Autodesk Inventor part; units mm, degrees
(part 2 of 3)
  line L262 (-273.1274, 163.0972) -> (-274.8776, 163.4871)
  line L263 (-274.8776, 163.4871) -> (-276.0608, 161.4819)
  line L264 (-276.0608, 161.4819) -> (-274.8734, 160.1383)
  line L265 (-274.8734, 160.1383) -> (-275.2904, 159.4316)
  line L266 (-275.5866, 163.6472) -> (-278.54, 164.2936)
  line L267 (-278.54, 164.2936) -> (-276.5438, 162.0252)
  line L268 (-276.5438, 162.0252) -> (-275.5866, 163.6472)
  line L269 (-271.6069, 165.6091) -> (-276.1953, 168.4149)
  line L270 (-276.1953, 168.4149) -> (-277.263, 166.669)
  line L271 (-277.263, 166.669) -> (-277.8787, 167.0455)
  line L272 (-277.8787, 167.0455) -> (-275.3204, 171.229)
  line L273 (-275.3204, 171.229) -> (-274.7047, 170.8525)
  line L274 (-274.7047, 170.8525) -> (-275.7724, 169.1065)
  line L275 (-275.7724, 169.1065) -> (-271.184, 166.3007)
  line L276 (-271.184, 166.3007) -> (-271.6069, 165.6091)
  spline S181 degree 2 poles (-268.782, 169.9517) (-269.136, 169.3919) (-269.8667, 168.7544) (-270.2531, 168.5133) knots 0 0 0 1 2 2 2
  line L277 (-270.2531, 168.5133) -> (-271.1138, 169.0576)
  line L278 (-271.1138, 169.0576) -> (-271.0821, 169.1077)
  spline S182 degree 2 poles (-271.0821, 169.1077) (-270.5505, 169.2453) (-269.6579, 169.8799) (-269.407, 170.2768) knots 0 0 0 1 2 2 2
  spline S183 degree 2 poles (-269.407, 170.2768) (-269.0476, 170.845) (-269.1525, 171.7243) (-269.541, 171.97) knots 0 0 0 1 2 2 2
  spline S184 degree 2 poles (-269.541, 171.97) (-269.8502, 172.1655) (-270.4275, 172.1036) (-270.7323, 171.8343) knots 0 0 0 1 2 2 2
  spline S185 degree 2 poles (-270.7323, 171.8343) (-270.9497, 171.6384) (-271.2926, 171.2996) (-271.5554, 171.0506) knots 0 0 0 1 2 2 2
  spline S186 degree 2 poles (-271.5554, 171.0506) (-271.7955, 170.8281) (-272.2755, 170.5408) (-272.5498, 170.4862) knots 0 0 0 1 2 2 2
  spline S187 degree 2 poles (-272.5498, 170.4862) (-272.8215, 170.4358) (-273.392, 170.5509) (-273.6929, 170.7412) knots 0 0 0 1 2 2 2
  spline S188 degree 2 poles (-273.6929, 170.7412) (-274.3196, 171.1375) (-274.5494, 172.6515) (-274.0712, 173.4077) knots 0 0 0 1 2 2 2
  spline S189 degree 2 poles (-274.0712, 173.4077) (-273.7964, 173.8422) (-273.139, 174.5026) (-272.7673, 174.7296) knots 0 0 0 1 2 2 2
  line L279 (-272.7673, 174.7296) -> (-271.9485, 174.2118)
  line L280 (-271.9485, 174.2118) -> (-271.9802, 174.1617)
  spline S190 degree 2 poles (-271.9802, 174.1617) (-272.3617, 174.0578) (-273.182, 173.5004) (-273.4489, 173.0785) knots 0 0 0 1 2 2 2
  spline S191 degree 2 poles (-273.4489, 173.0785) (-273.7501, 172.6022) (-273.6756, 171.7304) (-273.3121, 171.5005) knots 0 0 0 1 2 2 2
  spline S192 degree 2 poles (-273.3121, 171.5005) (-272.9862, 171.2944) (-272.3784, 171.3955) (-272.0845, 171.6659) knots 0 0 0 1 2 2 2
  spline S193 degree 2 poles (-272.0845, 171.6659) (-271.8887, 171.8462) (-271.3393, 172.3819) (-271.1445, 172.5512) knots 0 0 0 1 2 2 2
  spline S194 degree 2 poles (-271.1445, 172.5512) (-270.6461, 172.9788) (-269.6783, 173.057) (-269.1979, 172.7531) knots 0 0 0 1 2 2 2
  spline S195 degree 2 poles (-269.1979, 172.7531) (-268.8929, 172.5602) (-268.4639, 171.9439) (-268.3992, 171.593) knots 0 0 0 1 2 2 2
  spline S196 degree 2 poles (-268.3992, 171.593) (-268.3294, 171.2038) (-268.4834, 170.4239) (-268.782, 169.9517) knots 0 0 0 1 2 2 2
  line L281 (-267.6393, 171.9664) -> (-271.6185, 177.0265)
  line L282 (-271.6185, 177.0265) -> (-271.0719, 177.8622)
  line L283 (-271.0719, 177.8622) -> (-264.8413, 176.2439)
  line L284 (-264.8413, 176.2439) -> (-265.3095, 175.5282)
  line L285 (-265.3095, 175.5282) -> (-267.0398, 175.9985)
  line L286 (-267.0398, 175.9985) -> (-268.3143, 174.05)
  line L287 (-268.3143, 174.05) -> (-267.1901, 172.6531)
  line L288 (-267.1901, 172.6531) -> (-267.6393, 171.9664)
  line L289 (-267.7407, 176.1912) -> (-270.6611, 176.9732)
  line L290 (-270.6611, 176.9732) -> (-268.7717, 174.615)
  line L291 (-268.7717, 174.615) -> (-267.7407, 176.1912)
  spline S197 degree 2 poles (-266.5204, 183.3958) (-265.9906, 183.4543) (-264.7926, 183.1067) (-264.1628, 182.6789) knots 0 0 0 1 2 2 2
  spline S198 degree 2 poles (-264.1628, 182.6789) (-263.5494, 182.2623) (-262.7668, 181.2766) (-262.6315, 180.7545) knots 0 0 0 1 2 2 2
  spline S199 degree 2 poles (-262.6315, 180.7545) (-262.4909, 180.2048) (-262.7138, 179.1551) (-263.0499, 178.6603) knots 0 0 0 1 2 2 2
  spline S200 degree 2 poles (-263.0499, 178.6603) (-263.3971, 178.1492) (-264.3002, 177.5674) (-264.8423, 177.4994) knots 0 0 0 1 2 2 2
  spline S201 degree 2 poles (-264.8423, 177.4994) (-265.3748, 177.4368) (-266.5714, 177.7954) (-267.193, 178.2176) knots 0 0 0 1 2 2 2
  spline S202 degree 2 poles (-267.193, 178.2176) (-267.8268, 178.6481) (-268.578, 179.6184) (-268.7284, 180.1448) knots 0 0 0 1 2 2 2
  spline S203 degree 2 poles (-268.7284, 180.1448) (-268.8638, 180.667) (-268.6531, 181.725) (-268.3087, 182.2321) knots 0 0 0 1 2 2 2
  spline S204 degree 2 poles (-268.3087, 182.2321) (-267.9587, 182.7473) (-267.0378, 183.3289) (-266.5204, 183.3958) knots 0 0 0 1 2 2 2
  spline S205 degree 2 poles (-264.6378, 181.9797) (-265.1367, 182.3185) (-266.0567, 182.6267) (-266.4436, 182.6026) knots 0 0 0 1 2 2 2
  spline S206 degree 2 poles (-266.4436, 182.6026) (-266.8414, 182.58) (-267.4864, 182.1935) (-267.7252, 181.8418) knots 0 0 0 1 2 2 2
  spline S207 degree 2 poles (-267.7252, 181.8418) (-267.9724, 181.4778) (-268.0911, 180.7577) (-267.9628, 180.3658) knots 0 0 0 1 2 2 2
  spline S208 degree 2 poles (-267.9628, 180.3658) (-267.8413, 179.9905) (-267.2088, 179.2501) (-266.718, 178.9168) knots 0 0 0 1 2 2 2
  spline S209 degree 2 poles (-266.718, 178.9168) (-265.7244, 178.2419) (-264.1027, 178.3595) (-263.6278, 179.0588) knots 0 0 0 1 2 2 2
  spline S210 degree 2 poles (-263.6278, 179.0588) (-263.1529, 179.7581) (-263.6441, 181.3048) (-264.6378, 181.9797) knots 0 0 0 1 2 2 2
  spline S211 degree 2 poles (-259.7955, 183.3604) (-260.1062, 182.9202) (-260.7982, 182.4284) (-261.1909, 182.3607) knots 0 0 0 1 2 2 2
  spline S212 degree 2 poles (-261.1909, 182.3607) (-261.6346, 182.2806) (-262.5127, 182.5797) (-263.0458, 182.9559) knots 0 0 0 1 2 2 2
  line L292 (-263.0458, 182.9559) -> (-266.1555, 185.1508)
  line L293 (-266.1555, 185.1508) -> (-265.6881, 185.8131)
  line L294 (-265.6881, 185.8131) -> (-262.5783, 183.6183)
  spline S213 degree 2 poles (-262.5783, 183.6183) (-262.231, 183.3731) (-261.6998, 183.1313) (-261.4216, 183.1226) knots 0 0 0 1 2 2 2
  spline S214 degree 2 poles (-261.4216, 183.1226) (-261.1256, 183.1133) (-260.5947, 183.4283) (-260.3609, 183.7595) knots 0 0 0 1 2 2 2
  spline S215 degree 2 poles (-260.3609, 183.7595) (-260.1415, 184.0705) (-260.0054, 184.7005) (-260.1132, 184.9763) knots 0 0 0 1 2 2 2
  spline S216 degree 2 poles (-260.1132, 184.9763) (-260.2147, 185.2355) (-260.6164, 185.6521) (-260.9516, 185.8887) knots 0 0 0 1 2 2 2
  line L295 (-260.9516, 185.8887) -> (-264.0775, 188.095)
  line L296 (-264.0775, 188.095) -> (-263.6101, 188.7573)
  line L297 (-263.6101, 188.7573) -> (-260.5003, 186.5625)
  spline S217 degree 2 poles (-260.5003, 186.5625) (-259.9793, 186.1947) (-259.3844, 185.4602) (-259.3181, 185.0141) knots 0 0 0 1 2 2 2
  spline S218 degree 2 poles (-259.3181, 185.0141) (-259.2521, 184.6105) (-259.4706, 183.8208) (-259.7955, 183.3604) knots 0 0 0 1 2 2 2
  line L298 (-255.3693, 189.7045) -> (-255.9067, 188.9707)
  line L299 (-255.9067, 188.9707) -> (-261.7448, 189.9005)
  line L300 (-261.7448, 189.9005) -> (-257.5013, 186.7931)
  line L301 (-257.5013, 186.7931) -> (-257.9481, 186.1829)
  line L302 (-257.9481, 186.1829) -> (-262.8697, 189.7868)
  line L303 (-262.8697, 189.7868) -> (-262.1892, 190.7161)
  line L304 (-262.1892, 190.7161) -> (-256.8411, 189.8449)
  line L305 (-256.8411, 189.8449) -> (-260.7377, 192.6983)
  line L306 (-260.7377, 192.6983) -> (-260.2908, 193.3085)
  line L307 (-260.2908, 193.3085) -> (-255.3693, 189.7045)
  line L308 (-253.3463, 192.3891) -> (-254.7684, 190.502)
  line L309 (-254.7684, 190.502) -> (-255.2658, 190.8768)
  line L310 (-255.2658, 190.8768) -> (-254.7987, 191.4967)
  line L311 (-254.7987, 191.4967) -> (-258.6755, 194.4181)
  line L312 (-258.6755, 194.4181) -> (-259.1426, 193.7983)
  line L313 (-259.1426, 193.7983) -> (-259.64, 194.1731)
  line L314 (-259.64, 194.1731) -> (-258.218, 196.0602)
  line L315 (-258.218, 196.0602) -> (-257.7205, 195.6853)
  line L316 (-257.7205, 195.6853) -> (-258.1876, 195.0655)
  line L317 (-258.1876, 195.0655) -> (-254.3108, 192.1441)
  line L318 (-254.3108, 192.1441) -> (-253.8438, 192.7639)
  line L319 (-253.8438, 192.7639) -> (-253.3463, 192.3891)
  spline S219 degree 2 poles (-252.2013, 198.8575) (-251.5411, 198.3456) (-250.8937, 196.9864) (-250.9452, 196.307) knots 0 0 0 1 2 2 2
  spline S220 degree 2 poles (-250.9452, 196.307) (-250.9995, 195.761) (-251.4279, 194.886) (-251.8823, 194.3) knots 0 0 0 1 2 2 2
  line L320 (-251.8823, 194.3) -> (-252.7427, 193.1907)
  line L321 (-252.7427, 193.1907) -> (-257.563, 196.9289)
  line L322 (-257.563, 196.9289) -> (-256.7117, 198.0266)
  spline S221 degree 2 poles (-256.7117, 198.0266) (-256.1846, 198.7063) (-255.3816, 199.3222) (-254.9899, 199.4563) knots 0 0 0 1 2 2 2
  spline S222 degree 2 poles (-254.9899, 199.4563) (-254.3208, 199.6818) (-252.9044, 199.4028) (-252.2013, 198.8575) knots 0 0 0 1 2 2 2
  spline S223 degree 2 poles (-252.7271, 198.1956) (-253.2818, 198.6258) (-254.3517, 198.8675) (-254.8561, 198.6769) knots 0 0 0 1 2 2 2
  spline S224 degree 2 poles (-254.8561, 198.6769) (-255.2084, 198.5373) (-255.7965, 198.0613) (-256.1328, 197.6277) knots 0 0 0 1 2 2 2
  line L323 (-256.1328, 197.6277) -> (-256.5115, 197.1394)
  line L324 (-256.5115, 197.1394) -> (-252.8005, 194.2615)
  line L325 (-252.8005, 194.2615) -> (-252.4219, 194.7497)
  spline S225 degree 2 poles (-252.4219, 194.7497) (-252.0916, 195.1755) (-251.7285, 195.9261) (-251.7091, 196.3302) knots 0 0 0 1 2 2 2
  spline S226 degree 2 poles (-251.7091, 196.3302) (-251.6752, 196.8418) (-252.1646, 197.7594) (-252.7271, 198.1956) knots 0 0 0 1 2 2 2
  line L326 (-247.9163, 199.3374) -> (-249.3901, 197.4905)
  line L327 (-249.3901, 197.4905) -> (-249.877, 197.879)
  line L328 (-249.877, 197.879) -> (-249.3929, 198.4856)
  line L329 (-249.3929, 198.4856) -> (-253.1872, 201.5133)
  line L330 (-253.1872, 201.5133) -> (-253.6713, 200.9067)
  line L331 (-253.6713, 200.9067) -> (-254.1582, 201.2952)
  line L332 (-254.1582, 201.2952) -> (-252.6844, 203.1421)
  line L333 (-252.6844, 203.1421) -> (-252.1975, 202.7537)
  line L334 (-252.1975, 202.7537) -> (-252.6816, 202.147)
  line L335 (-252.6816, 202.147) -> (-248.8873, 199.1193)
  line L336 (-248.8873, 199.1193) -> (-248.4032, 199.7259)
  line L337 (-248.4032, 199.7259) -> (-247.9163, 199.3374)
  spline S227 degree 2 poles (-246.1272, 201.3672) (-246.5467, 200.8545) (-247.3494, 200.3106) (-247.7623, 200.1183) knots 0 0 0 1 2 2 2
  line L338 (-247.7623, 200.1183) -> (-248.5504, 200.7631)
  line L339 (-248.5504, 200.7631) -> (-248.5128, 200.809)
  spline S228 degree 2 poles (-248.5128, 200.809) (-247.9685, 200.881) (-247.0054, 201.4023) (-246.708, 201.7658) knots 0 0 0 1 2 2 2
  spline S229 degree 2 poles (-246.708, 201.7658) (-246.2823, 202.2861) (-246.2795, 203.1716) (-246.6353, 203.4627) knots 0 0 0 1 2 2 2
  spline S230 degree 2 poles (-246.6353, 203.4627) (-246.9184, 203.6944) (-247.4989, 203.7031) (-247.8342, 203.4729) knots 0 0 0 1 2 2 2
  spline S231 degree 2 poles (-247.8342, 203.4729) (-248.0738, 203.3049) (-248.4554, 203.0103) (-248.7465, 202.795) knots 0 0 0 1 2 2 2
  spline S232 degree 2 poles (-248.7465, 202.795) (-249.0119, 202.6034) (-249.5232, 202.3766) (-249.8021, 202.3558) knots 0 0 0 1 2 2 2
  spline S233 degree 2 poles (-249.8021, 202.3558) (-250.0779, 202.3387) (-250.6302, 202.5224) (-250.9057, 202.7478) knots 0 0 0 1 2 2 2
  spline S234 degree 2 poles (-250.9057, 202.7478) (-251.4796, 203.2173) (-251.5237, 204.748) (-250.9571, 205.4405) knots 0 0 0 1 2 2 2
  spline S235 degree 2 poles (-250.9571, 205.4405) (-250.6315, 205.8384) (-249.8987, 206.414) (-249.5022, 206.5941) knots 0 0 0 1 2 2 2
  line L340 (-249.5022, 206.5941) -> (-248.7523, 205.9806)
  line L341 (-248.7523, 205.9806) -> (-248.7899, 205.9347)
  spline S236 degree 2 poles (-248.7899, 205.9347) (-249.1812, 205.878) (-250.0632, 205.4245) (-250.3794, 205.0381) knots 0 0 0 1 2 2 2
  spline S237 degree 2 poles (-250.3794, 205.0381) (-250.7362, 204.6019) (-250.7683, 203.7276) (-250.4354, 203.4552) knots 0 0 0 1 2 2 2
  spline S238 degree 2 poles (-250.4354, 203.4552) (-250.137, 203.211) (-249.5214, 203.2375) (-249.1969, 203.4701) knots 0 0 0 1 2 2 2
  spline S239 degree 2 poles (-249.1969, 203.4701) (-248.9805, 203.6252) (-248.3701, 204.0902) (-248.1562, 204.2346) knots 0 0 0 1 2 2 2
  spline S240 degree 2 poles (-248.1562, 204.2346) (-247.6095, 204.5984) (-246.6394, 204.5583) (-246.1995, 204.1983) knots 0 0 0 1 2 2 2
  spline S241 degree 2 poles (-246.1995, 204.1983) (-245.9202, 203.9698) (-245.5693, 203.3059) (-245.5477, 202.9497) knots 0 0 0 1 2 2 2
  spline S242 degree 2 poles (-245.5477, 202.9497) (-245.5258, 202.5549) (-245.7735, 201.7995) (-246.1272, 201.3672) knots 0 0 0 1 2 2 2
  spline S243 degree 2 poles (-241.7417, 209.8177) (-241.3851, 209.5121) (-240.9834, 208.7578) (-240.9512, 208.3851) knots 0 0 0 1 2 2 2
  spline S244 degree 2 poles (-240.9512, 208.3851) (-240.9142, 207.9953) (-241.1366, 207.2876) (-241.4036, 206.976) knots 0 0 0 1 2 2 2
  spline S245 degree 2 poles (-241.4036, 206.976) (-241.6706, 206.6645) (-242.3215, 206.3304) (-242.6989, 206.3153) knots 0 0 0 1 2 2 2
  spline S246 degree 2 poles (-242.6989, 206.3153) (-243.1563, 206.2906) (-244.2324, 206.7441) (-244.848, 207.2717) knots 0 0 0 1 2 2 2
  spline S247 degree 2 poles (-244.848, 207.2717) (-245.4523, 207.7895) (-246.2122, 208.8704) (-246.3506, 209.4382) knots 0 0 0 1 2 2 2
  spline S248 degree 2 poles (-246.3506, 209.4382) (-246.4879, 209.9921) (-246.2001, 211.1255) (-245.753, 211.6473) knots 0 0 0 1 2 2 2
  spline S249 degree 2 poles (-245.753, 211.6473) (-245.6211, 211.8012) (-245.3594, 212.0457) (-245.2388, 212.1181) knots 0 0 0 1 2 2 2
  line L342 (-245.2388, 212.1181) -> (-244.642, 211.6066)
  line L343 (-244.642, 211.6066) -> (-244.6645, 211.5804)
  spline S250 degree 2 poles (-244.6645, 211.5804) (-244.7835, 211.5326) (-245.1326, 211.2849) (-245.287, 211.1047) knots 0 0 0 1 2 2 2
  spline S251 degree 2 poles (-245.287, 211.1047) (-245.7823, 210.5267) (-245.6096, 209.1482) (-244.9017, 208.4244) knots 0 0 0 1 2 2 2
  spline S252 degree 2 poles (-244.9017, 208.4244) (-244.8659, 208.7778) (-244.6359, 209.388) (-244.3979, 209.6657) knots 0 0 0 1 2 2 2
  spline S253 degree 2 poles (-244.3979, 209.6657) (-244.1663, 209.936) (-243.71, 210.2481) (-243.3551, 210.328) knots 0 0 0 1 2 2 2
  spline S254 degree 2 poles (-243.3551, 210.328) (-242.9449, 210.4192) (-242.1395, 210.1587) (-241.7417, 209.8177) knots 0 0 0 1 2 2 2
  spline S255 degree 2 poles (-242.2558, 209.1646) (-242.5411, 209.4091) (-243.0563, 209.5902) (-243.333, 209.5409) knots 0 0 0 1 2 2 2
  spline S256 degree 2 poles (-243.333, 209.5409) (-243.5367, 209.5007) (-243.8643, 209.2476) (-244.0026, 209.0861) knots 0 0 0 1 2 2 2
  spline S257 degree 2 poles (-244.0026, 209.0861) (-244.1892, 208.8684) (-244.4085, 208.3467) (-244.4551, 208.0416) knots 0 0 0 1 2 2 2
  spline S258 degree 2 poles (-244.4551, 208.0416) (-244.3907, 207.98) (-244.2695, 207.8631) (-244.172, 207.7795) knots 0 0 0 1 2 2 2
  spline S259 degree 2 poles (-244.172, 207.7795) (-243.6915, 207.3677) (-242.9414, 207.0504) (-242.6652, 207.0611) knots 0 0 0 1 2 2 2
  spline S260 degree 2 poles (-242.6652, 207.0611) (-242.4063, 207.0671) (-242.0454, 207.2526) (-241.9071, 207.414) knots 0 0 0 1 2 2 2
  spline S261 degree 2 poles (-241.9071, 207.414) (-241.5855, 207.7894) (-241.7228, 208.7078) (-242.2558, 209.1646) knots 0 0 0 1 2 2 2
  spline S262 degree 2 poles (-242.8173, 213.9622) (-242.9645, 213.7954) (-243.174, 213.3935) (-243.2516, 213.1786) knots 0 0 0 1 2 2 2
  spline S263 degree 2 poles (-243.2516, 213.1786) (-243.3194, 212.9747) (-243.3789, 212.6383) (-243.3948, 212.5007) knots 0 0 0 1 2 2 2
  line L344 (-243.3948, 212.5007) -> (-243.4275, 212.4636)
  line L345 (-243.4275, 212.4636) -> (-244.0762, 213.0359)
  spline S264 degree 2 poles (-244.0762, 213.0359) (-244.0071, 213.3309) (-243.5763, 214.1704) (-243.3049, 214.4781) knots 0 0 0 1 2 2 2
  spline S265 degree 2 poles (-243.3049, 214.4781) (-243.0302, 214.7894) (-242.4953, 215.1416) (-242.1951, 215.2129) knots 0 0 0 1 2 2 2
  spline S266 degree 2 poles (-242.1951, 215.2129) (-241.8739, 215.2855) (-241.2719, 215.1236) (-240.9902, 214.875) knots 0 0 0 1 2 2 2
  spline S267 degree 2 poles (-240.9902, 214.875) (-240.6121, 214.5414) (-240.4795, 213.5411) (-240.7127, 213.1272) knots 0 0 0 1 2 2 2
  line L346 (-240.7127, 213.1272) -> (-240.6683, 213.088)
  spline S268 degree 2 poles (-240.6683, 213.088) (-240.5111, 213.2064) (-240.0866, 213.4186) (-239.8288, 213.4417) knots 0 0 0 1 2 2 2
  spline S269 degree 2 poles (-239.8288, 213.4417) (-239.5748, 213.4681) (-239.0027, 213.2798) (-238.7024, 213.0149) knots 0 0 0 1 2 2 2
  spline S270 degree 2 poles (-238.7024, 213.0149) (-238.3948, 212.7434) (-238.0585, 212.071) (-238.0284, 211.7016) knots 0 0 0 1 2 2 2
  spline S271 degree 2 poles (-238.0284, 211.7016) (-237.9974, 211.3183) (-238.2828, 210.5615) (-238.6, 210.2019) knots 0 0 0 1 2 2 2
  spline S272 degree 2 poles (-238.6, 210.2019) (-238.9042, 209.8572) (-239.6662, 209.3297) (-239.9838, 209.2013) knots 0 0 0 1 2 2 2
  line L347 (-239.9838, 209.2013) -> (-240.6325, 209.7736)
  line L348 (-240.6325, 209.7736) -> (-240.5933, 209.8181)
  spline S273 degree 2 poles (-240.5933, 209.8181) (-240.2824, 209.8866) (-239.4473, 210.31) (-239.1628, 210.6325) knots 0 0 0 1 2 2 2
  spline S274 degree 2 poles (-239.1628, 210.6325) (-238.996, 210.8216) (-238.781, 211.3043) (-238.807, 211.5514) knots 0 0 0 1 2 2 2
  spline S275 degree 2 poles (-238.807, 211.5514) (-238.8362, 211.7947) (-239.048, 212.2122) (-239.2963, 212.4313) knots 0 0 0 1 2 2 2
  spline S276 degree 2 poles (-239.2963, 212.4313) (-239.5447, 212.6505) (-239.9947, 212.7904) (-240.2019, 212.7424) knots 0 0 0 1 2 2 2
  spline S277 degree 2 poles (-240.2019, 212.7424) (-240.409, 212.6945) (-240.7901, 212.4044) (-240.9733, 212.1969) knots 0 0 0 1 2 2 2
  line L349 (-240.9733, 212.1969) -> (-241.2022, 211.9374)
  line L350 (-241.2022, 211.9374) -> (-241.71, 212.3854)
  line L351 (-241.71, 212.3854) -> (-241.5301, 212.5893)
  spline S278 degree 2 poles (-241.5301, 212.5893) (-241.1671, 213.0008) (-241.1022, 213.8664) (-241.4766, 214.1967) knots 0 0 0 1 2 2 2
  spline S279 degree 2 poles (-241.4766, 214.1967) (-241.6508, 214.3504) (-242.0169, 214.4361) (-242.1859, 214.394) knots 0 0 0 1 2 2 2
  spline S280 degree 2 poles (-242.1859, 214.394) (-242.3651, 214.3477) (-242.6767, 214.1216) (-242.8173, 213.9622) knots 0 0 0 1 2 2 2
  line L352 (-234.2036, 215.2879) -> (-236.7327, 212.5031)
  line L353 (-236.7327, 212.5031) -> (-237.3731, 213.0847)
  spline S281 degree 2 poles (-237.3731, 213.0847) (-237.3823, 213.6407) (-237.4204, 214.6502) (-237.4695, 215.1622) knots 0 0 0 1 2 2 2
  spline S282 degree 2 poles (-237.4695, 215.1622) (-237.5682, 216.1933) (-237.9065, 217.1884) (-238.2688, 217.5174) knots 0 0 0 1 2 2 2
  spline S283 degree 2 poles (-238.2688, 217.5174) (-238.4591, 217.6902) (-238.8508, 217.8323) (-239.0387, 217.8093) knots 0 0 0 1 2 2 2
  spline S284 degree 2 poles (-239.0387, 217.8093) (-239.2266, 217.7863) (-239.5706, 217.5912) (-239.7235, 217.4229) knots 0 0 0 1 2 2 2
  spline S285 degree 2 poles (-239.7235, 217.4229) (-239.8697, 217.2619) (-240.0883, 216.8594) (-240.1624, 216.6529) knots 0 0 0 1 2 2 2
  spline S286 degree 2 poles (-240.1624, 216.6529) (-240.2275, 216.4783) (-240.2971, 216.1075) (-240.3123, 215.9878) knots 0 0 0 1 2 2 2
  line L354 (-240.3123, 215.9878) -> (-240.3423, 215.9548)
  line L355 (-240.3423, 215.9548) -> (-240.9863, 216.5398)
  spline S287 degree 2 poles (-240.9863, 216.5398) (-240.9083, 216.8095) (-240.4794, 217.642) (-240.2069, 217.9421) knots 0 0 0 1 2 2 2
  spline S288 degree 2 poles (-240.2069, 217.9421) (-239.632, 218.5751) (-238.3143, 218.6805) (-237.7434, 218.1621) knots 0 0 0 1 2 2 2
  spline S289 degree 2 poles (-237.7434, 218.1621) (-237.4762, 217.9195) (-237.1428, 217.3896) (-237.0522, 217.107) knots 0 0 0 1 2 2 2
  spline S290 degree 2 poles (-237.0522, 217.107) (-236.9543, 216.8178) (-236.8555, 216.1471) (-236.8284, 215.802) knots 0 0 0 1 2 2 2
  spline S291 degree 2 poles (-236.8284, 215.802) (-236.7766, 215.2341) (-236.7454, 213.9303) (-236.7408, 213.5455) knots 0 0 0 1 2 2 2
  line L356 (-236.7408, 213.5455) -> (-234.7269, 215.7631)
  line L357 (-234.7269, 215.7631) -> (-234.2036, 215.2879)
  spline S292 degree 2 poles (-232.2903, 217.1398) (-232.6008, 216.8076) (-233.3092, 216.448) (-233.6723, 216.4287) knots 0 0 0 1 2 2 2
  spline S293 degree 2 poles (-233.6723, 216.4287) (-234.0284, 216.4097) (-234.7018, 216.6738) (-234.9798, 216.9337) knots 0 0 0 1 2 2 2
  spline S294 degree 2 poles (-234.9798, 216.9337) (-235.341, 217.2713) (-235.5864, 218.2248) (-235.4227, 218.762) knots 0 0 0 1 2 2 2
  line L358 (-235.4227, 218.762) -> (-235.4407, 218.7788)
  spline S295 degree 2 poles (-235.4407, 218.7788) (-235.9393, 218.6291) (-236.6914, 218.7367) (-237.0308, 219.054) knots 0 0 0 1 2 2 2
  spline S296 degree 2 poles (-237.0308, 219.054) (-237.5328, 219.5232) (-237.4956, 220.9094) (-236.9487, 221.4944) knots 0 0 0 1 2 2 2
  spline S297 degree 2 poles (-236.9487, 221.4944) (-236.3816, 222.1011) (-235.0608, 222.2401) (-234.5624, 221.7742) knots 0 0 0 1 2 2 2
  spline S298 degree 2 poles (-234.5624, 221.7742) (-234.2627, 221.4941) (-234.0051, 220.5969) (-234.1462, 220.113) knots 0 0 0 1 2 2 2
  line L359 (-234.1462, 220.113) -> (-234.1282, 220.0961)
  spline S299 degree 2 poles (-234.1282, 220.0961) (-233.583, 220.3174) (-232.6883, 220.2321) (-232.2766, 219.8473) knots 0 0 0 1 2 2 2
  spline S300 degree 2 poles (-232.2766, 219.8473) (-231.7061, 219.3139) (-231.7097, 217.761) (-232.2903, 217.1398) knots 0 0 0 1 2 2 2
  spline S301 degree 2 poles (-232.7927, 219.1794) (-233.0672, 219.4359) (-233.5947, 219.5231) (-234.0478, 219.3714) knots 0 0 0 1 2 2 2
  spline S302 degree 2 poles (-234.0478, 219.3714) (-234.2001, 219.3243) (-234.651, 219.1097) (-234.9368, 218.9777) knots 0 0 0 1 2 2 2
  spline S303 degree 2 poles (-234.9368, 218.9777) (-235.0039, 218.5802) (-234.7664, 217.8643) (-234.4594, 217.5773) knots 0 0 0 1 2 2 2
  spline S304 degree 2 poles (-234.4594, 217.5773) (-234.055, 217.1993) (-233.072, 217.1939) (-232.7277, 217.5623) knots 0 0 0 1 2 2 2
  spline S305 degree 2 poles (-232.7277, 217.5623) (-232.3766, 217.9378) (-232.4027, 218.8148) (-232.7927, 219.1794) knots 0 0 0 1 2 2 2
  spline S306 degree 2 poles (-235.1021, 221.1825) (-235.4018, 221.4627) (-236.1774, 221.4365) (-236.5115, 221.079) knots 0 0 0 1 2 2 2
  spline S307 degree 2 poles (-236.5115, 221.079) (-236.8154, 220.754) (-236.846, 220.0045) (-236.5391, 219.7176) knots 0 0 0 1 2 2 2
  spline S308 degree 2 poles (-236.5391, 219.7176) (-236.3188, 219.5117) (-235.8127, 219.4378) (-235.4908, 219.5361) knots 0 0 0 1 2 2 2
  spline S309 degree 2 poles (-235.4908, 219.5361) (-235.3558, 219.5791) (-234.821, 219.7965) (-234.6253, 219.9045) knots 0 0 0 1 2 2 2
  spline S310 degree 2 poles (-234.6253, 219.9045) (-234.5809, 220.3502) (-234.8312, 220.9293) (-235.1021, 221.1825) knots 0 0 0 1 2 2 2
  line L360 (-225.3795, 224.5158) -> (-228.2028, 230.3009)
  line L361 (-228.2028, 230.3009) -> (-227.4923, 231.0026)
  line L362 (-227.4923, 231.0026) -> (-221.7428, 228.1074)
  line L363 (-221.7428, 228.1074) -> (-222.3513, 227.5065)
  line L364 (-222.3513, 227.5065) -> (-223.9436, 228.3309)
  line L365 (-223.9436, 228.3309) -> (-225.6001, 226.6948)
  line L366 (-225.6001, 226.6948) -> (-224.7957, 225.0924)
  line L367 (-224.7957, 225.0924) -> (-225.3795, 224.5158)
  line L368 (-224.5881, 228.667) -> (-227.278, 230.047)
  line L369 (-227.278, 230.047) -> (-225.9282, 227.3435)
  line L370 (-225.9282, 227.3435) -> (-224.5881, 228.667)
  line L371 (-218.1124, 231.5778) -> (-218.7702, 230.9497)
  line L372 (-218.7702, 230.9497) -> (-224.3545, 232.8897)
  line L373 (-224.3545, 232.8897) -> (-220.7222, 229.0857)
  line L374 (-220.7222, 229.0857) -> (-221.2692, 228.5634)
  line L375 (-221.2692, 228.5634) -> (-225.4819, 232.9751)
  line L376 (-225.4819, 232.9751) -> (-224.6489, 233.7705)
  line L377 (-224.6489, 233.7705) -> (-219.5367, 231.9743)
  line L378 (-219.5367, 231.9743) -> (-222.872, 235.4672)
  line L379 (-222.872, 235.4672) -> (-222.325, 235.9895)
  line L380 (-222.325, 235.9895) -> (-218.1124, 231.5778)
  spline S311 degree 2 poles (-215.2516, 234.0683) (-215.7277, 233.6294) (-216.7845, 233.1931) (-217.3394, 233.2262) knots 0 0 0 1 2 2 2
  spline S312 degree 2 poles (-217.3394, 233.2262) (-217.8976, 233.2629) (-219.0101, 233.8644) (-219.5361, 234.4351) knots 0 0 0 1 2 2 2
  spline S313 degree 2 poles (-219.5361, 234.4351) (-220.0353, 234.9766) (-220.5207, 236.1158) (-220.5186, 236.6825) knots 0 0 0 1 2 2 2
  spline S314 degree 2 poles (-220.5186, 236.6825) (-220.5174, 237.2282) (-220.0126, 238.2851) (-219.5364, 238.724) knots 0 0 0 1 2 2 2
  spline S315 degree 2 poles (-219.5364, 238.724) (-219.3074, 238.9351) (-218.8328, 239.2516) (-218.5902, 239.3677) knots 0 0 0 1 2 2 2
  spline S316 degree 2 poles (-218.5902, 239.3677) (-218.3973, 239.4648) (-217.8792, 239.6466) (-217.7129, 239.6923) knots 0 0 0 1 2 2 2
  line L381 (-217.7129, 239.6923) -> (-217.0495, 238.9726)
  line L382 (-217.0495, 238.9726) -> (-217.1004, 238.9257)
  spline S317 degree 2 poles (-217.1004, 238.9257) (-217.3035, 238.92) (-217.7039, 238.8803) (-218.0158, 238.7811) knots 0 0 0 1 2 2 2
  spline S318 degree 2 poles (-218.0158, 238.7811) (-218.2813, 238.7044) (-218.8608, 238.3922) (-219.1297, 238.1442) knots 0 0 0 1 2 2 2
  spline S319 degree 2 poles (-219.1297, 238.1442) (-219.7767, 237.5479) (-219.6784, 235.8367) (-218.9313, 235.0261) knots 0 0 0 1 2 2 2
  spline S320 degree 2 poles (-218.9313, 235.0261) (-218.5159, 234.5754) (-217.6819, 234.0937) (-217.2675, 234.0454) knots 0 0 0 1 2 2 2
  spline S321 degree 2 poles (-217.2675, 234.0454) (-216.8605, 233.9903) (-216.0908, 234.2494) (-215.7491, 234.5643) knots 0 0 0 1 2 2 2
  spline S322 degree 2 poles (-215.7491, 234.5643) (-215.4984, 234.7955) (-215.0638, 235.3305) (-214.9599, 235.5607) knots 0 0 0 1 2 2 2
  line L383 (-214.9599, 235.5607) -> (-216.0287, 236.7201)
  line L384 (-216.0287, 236.7201) -> (-217.0682, 235.7619)
  line L385 (-217.0682, 235.7619) -> (-217.5507, 236.2853)
  line L386 (-217.5507, 236.2853) -> (-215.9224, 237.7863)
  line L387 (-215.9224, 237.7863) -> (-214.1165, 235.8272)
  spline S323 degree 2 poles (-214.1165, 235.8272) (-214.1823, 235.6724) (-214.4235, 235.161) (-214.5435, 234.963) knots 0 0 0 1 2 2 2
  spline S324 degree 2 poles (-214.5435, 234.963) (-214.7049, 234.6932) (-215.0008, 234.2994) (-215.2516, 234.0683) knots 0 0 0 1 2 2 2
  line L388 (-213.0839, 236.2092) -> (-217.145, 240.7608)
  line L389 (-217.145, 240.7608) -> (-214.2975, 243.3015)
  line L390 (-214.2975, 243.3015) -> (-213.817, 242.763)
  line L391 (-213.817, 242.763) -> (-216.0596, 240.762)
  line L392 (-216.0596, 240.762) -> (-214.9473, 239.5153)
  line L393 (-214.9473, 239.5153) -> (-212.8559, 241.3814)
  line L394 (-212.8559, 241.3814) -> (-212.3754, 240.8428)
  line L395 (-212.3754, 240.8428) -> (-214.4668, 238.9768)
  line L396 (-214.4668, 238.9768) -> (-212.9595, 237.2875)
  line L397 (-212.9595, 237.2875) -> (-210.7169, 239.2884)
  line L398 (-210.7169, 239.2884) -> (-210.2364, 238.7499)
  line L399 (-210.2364, 238.7499) -> (-213.0839, 236.2092)
  line L400 (-206.8957, 241.6505) -> (-209.5655, 239.3344)
  line L401 (-209.5655, 239.3344) -> (-213.5628, 243.9423)
  line L402 (-213.5628, 243.9423) -> (-212.9504, 244.4735)
  line L403 (-212.9504, 244.4735) -> (-209.4261, 240.4109)
  line L404 (-209.4261, 240.4109) -> (-207.3686, 242.1957)
  line L405 (-207.3686, 242.1957) -> (-206.8957, 241.6505)
  spline S325 degree 2 poles (-206.5831, 248.979) (-206.0574, 248.8912) (-204.9991, 248.2308) (-204.5094, 247.6479) knots 0 0 0 1 2 2 2
  spline S326 degree 2 poles (-204.5094, 247.6479) (-204.0325, 247.0802) (-203.5475, 245.9188) (-203.5593, 245.3795) knots 0 0 0 1 2 2 2
  spline S327 degree 2 poles (-203.5593, 245.3795) (-203.5735, 244.8123) (-204.0736, 243.8628) (-204.5316, 243.4781) knots 0 0 0 1 2 2 2
  spline S328 degree 2 poles (-204.5316, 243.4781) (-205.0047, 243.0807) (-206.032, 242.7665) (-206.5722, 242.8485) knots 0 0 0 1 2 2 2
  spline S329 degree 2 poles (-206.5722, 242.8485) (-207.1017, 242.9332) (-208.1556, 243.6037) (-208.6389, 244.179) knots 0 0 0 1 2 2 2
  spline S330 degree 2 poles (-208.6389, 244.179) (-209.1317, 244.7657) (-209.5906, 245.9038) (-209.5922, 246.4513) knots 0 0 0 1 2 2 2
  spline S331 degree 2 poles (-209.5922, 246.4513) (-209.5804, 246.9906) (-209.0898, 247.9514) (-208.6205, 248.3457) knots 0 0 0 1 2 2 2
  spline S332 degree 2 poles (-208.6205, 248.3457) (-208.1436, 248.7463) (-207.0992, 249.0555) (-206.5831, 248.979) knots 0 0 0 1 2 2 2
  spline S333 degree 2 poles (-205.1567, 247.1042) (-205.5446, 247.566) (-206.3461, 248.1129) (-206.7249, 248.1949) knots 0 0 0 1 2 2 2
  spline S334 degree 2 poles (-206.7249, 248.1949) (-207.1139, 248.2814) (-207.8397, 248.0848) (-208.1652, 247.8114) knots 0 0 0 1 2 2 2
  spline S335 degree 2 poles (-208.1652, 247.8114) (-208.5021, 247.5284) (-208.8121, 246.8677) (-208.7953, 246.4557) knots 0 0 0 1 2 2 2
  spline S336 degree 2 poles (-208.7953, 246.4557) (-208.7805, 246.0614) (-208.3732, 245.177) (-207.9916, 244.7227) knots 0 0 0 1 2 2 2
  spline S337 degree 2 poles (-207.9916, 244.7227) (-207.219, 243.803) (-205.6266, 243.4751) (-204.9793, 244.0188) knots 0 0 0 1 2 2 2
  spline S338 degree 2 poles (-204.9793, 244.0188) (-204.3321, 244.5625) (-204.384, 246.1845) (-205.1567, 247.1042) knots 0 0 0 1 2 2 2
  spline S339 degree 2 poles (-200.4678, 246.8603) (-200.982, 246.4428) (-201.8779, 246.0719) (-202.3211, 245.9668) knots 0 0 0 1 2 2 2
  line L406 (-202.3211, 245.9668) -> (-202.963, 246.7573)
  line L407 (-202.963, 246.7573) -> (-202.9169, 246.7947)
  spline S340 degree 2 poles (-202.9169, 246.7947) (-202.3693, 246.7554) (-201.3208, 247.0718) (-200.9563, 247.3679) knots 0 0 0 1 2 2 2
  spline S341 degree 2 poles (-200.9563, 247.3679) (-200.4344, 247.7916) (-200.2531, 248.6584) (-200.5429, 249.0153) knots 0 0 0 1 2 2 2
  spline S342 degree 2 poles (-200.5429, 249.0153) (-200.7734, 249.2993) (-201.3402, 249.4249) (-201.7151, 249.267) knots 0 0 0 1 2 2 2
  spline S343 degree 2 poles (-201.7151, 249.267) (-201.9837, 249.1507) (-202.4168, 248.9392) (-202.7453, 248.787) knots 0 0 0 1 2 2 2
  spline S344 degree 2 poles (-202.7453, 248.787) (-203.0439, 248.6528) (-203.5904, 248.5338) (-203.8678, 248.5696) knots 0 0 0 1 2 2 2
  spline S345 degree 2 poles (-203.8678, 248.5696) (-204.1414, 248.6085) (-204.6454, 248.8998) (-204.8697, 249.1761) knots 0 0 0 1 2 2 2
  spline S346 degree 2 poles (-204.8697, 249.1761) (-205.3371, 249.7517) (-205.0717, 251.2599) (-204.3771, 251.8239) knots 0 0 0 1 2 2 2
  spline S347 degree 2 poles (-204.3771, 251.8239) (-203.978, 252.148) (-203.1441, 252.564) (-202.7194, 252.6605) knots 0 0 0 1 2 2 2
  line L408 (-202.7194, 252.6605) -> (-202.1087, 251.9083)
  line L409 (-202.1087, 251.9083) -> (-202.1547, 251.8709)
  spline S348 degree 2 poles (-202.1547, 251.8709) (-202.5494, 251.8943) (-203.5048, 251.628) (-203.8924, 251.3132) knots 0 0 0 1 2 2 2
  spline S349 degree 2 poles (-203.8924, 251.3132) (-204.3299, 250.958) (-204.5376, 250.108) (-204.2665, 249.7742) knots 0 0 0 1 2 2 2
  spline S350 degree 2 poles (-204.2665, 249.7742) (-204.0234, 249.4749) (-203.4151, 249.3766) (-203.0504, 249.539) knots 0 0 0 1 2 2 2
  spline S351 degree 2 poles (-203.0504, 249.539) (-202.8072, 249.6474) (-202.1155, 249.9797) (-201.8769, 250.078) knots 0 0 0 1 2 2 2
  spline S352 degree 2 poles (-201.8769, 250.078) (-201.268, 250.324) (-200.326, 250.0892) (-199.9677, 249.6479) knots 0 0 0 1 2 2 2
  spline S353 degree 2 poles (-199.9677, 249.6479) (-199.7402, 249.3678) (-199.5304, 248.6467) (-199.5811, 248.2935) knots 0 0 0 1 2 2 2
  spline S354 degree 2 poles (-199.5811, 248.2935) (-199.6392, 247.9024) (-200.0341, 247.2124) (-200.4678, 246.8603) knots 0 0 0 1 2 2 2
  spline S355 degree 2 poles (-194.7575, 251.3898) (-195.2812, 250.9842) (-196.1854, 250.6339) (-196.6308, 250.539) knots 0 0 0 1 2 2 2
  line L410 (-196.6308, 250.539) -> (-197.2544, 251.344)
  line L411 (-197.2544, 251.344) -> (-197.2076, 251.3803)
  spline S356 degree 2 poles (-197.2076, 251.3803) (-196.6609, 251.3285) (-195.6055, 251.6209) (-195.2343, 251.9084) knots 0 0 0 1 2 2 2
  spline S357 degree 2 poles (-195.2343, 251.9084) (-194.7028, 252.3201) (-194.5017, 253.1825) (-194.7832, 253.546) knots 0 0 0 1 2 2 2
  spline S358 degree 2 poles (-194.7832, 253.546) (-195.0072, 253.8352) (-195.571, 253.9737) (-195.9494, 253.8244) knots 0 0 0 1 2 2 2
  spline S359 degree 2 poles (-195.9494, 253.8244) (-196.2205, 253.7144) (-196.6584, 253.5128) (-196.9903, 253.3682) knots 0 0 0 1 2 2 2
  spline S360 degree 2 poles (-196.9903, 253.3682) (-197.2919, 253.2409) (-197.841, 253.1344) (-198.1175, 253.1766) knots 0 0 0 1 2 2 2
  spline S361 degree 2 poles (-198.1175, 253.1766) (-198.3901, 253.2218) (-198.8873, 253.5245) (-199.1052, 253.8059) knots 0 0 0 1 2 2 2
  spline S362 degree 2 poles (-199.1052, 253.8059) (-199.5593, 254.3921) (-199.2594, 255.8938) (-198.5521, 256.4417) knots 0 0 0 1 2 2 2
  spline S363 degree 2 poles (-198.5521, 256.4417) (-198.1456, 256.7565) (-197.3025, 257.1533) (-196.8757, 257.24) knots 0 0 0 1 2 2 2
  line L412 (-196.8757, 257.24) -> (-196.2823, 256.4741)
  line L413 (-196.2823, 256.4741) -> (-196.3292, 256.4378)
  spline S364 degree 2 poles (-196.3292, 256.4378) (-196.7233, 256.4702) (-197.6845, 256.2258) (-198.0792, 255.9201) knots 0 0 0 1 2 2 2
  spline S365 degree 2 poles (-198.0792, 255.9201) (-198.5247, 255.575) (-198.7518, 254.73) (-198.4884, 254.39) knots 0 0 0 1 2 2 2
  spline S366 degree 2 poles (-198.4884, 254.39) (-198.2523, 254.0852) (-197.6464, 253.973) (-197.278, 254.127) knots 0 0 0 1 2 2 2
  spline S367 degree 2 poles (-197.278, 254.127) (-197.0324, 254.2298) (-196.3334, 254.5462) (-196.0926, 254.6389) knots 0 0 0 1 2 2 2
  spline S368 degree 2 poles (-196.0926, 254.6389) (-195.4782, 254.871) (-194.5418, 254.6146) (-194.1937, 254.1652) knots 0 0 0 1 2 2 2
  spline S369 degree 2 poles (-194.1937, 254.1652) (-193.9727, 253.8799) (-193.7794, 253.1542) (-193.8382, 252.8023) knots 0 0 0 1 2 2 2
  spline S370 degree 2 poles (-193.8382, 252.8023) (-193.9053, 252.4127) (-194.3159, 251.7319) (-194.7575, 251.3898) knots 0 0 0 1 2 2 2
  line L414 (-191.3319, 254.1433) -> (-194.5611, 258.4442)
  line L415 (-194.5611, 258.4442) -> (-196.1977, 257.2154)
  line L416 (-196.1977, 257.2154) -> (-196.631, 257.7926)
  line L417 (-196.631, 257.7926) -> (-192.7096, 260.7369)
  line L418 (-192.7096, 260.7369) -> (-192.2763, 260.1597)
  line L419 (-192.2763, 260.1597) -> (-193.9128, 258.931)
  line L420 (-193.9128, 258.931) -> (-190.6836, 254.63)
  line L421 (-190.6836, 254.63) -> (-191.3319, 254.1433)
  line L422 (-188.5429, 256.2247) -> (-192.1314, 261.1575)
  line L423 (-192.1314, 261.1575) -> (-189.0454, 263.4025)
  line L424 (-189.0454, 263.4025) -> (-188.6209, 262.8189)
  line L425 (-188.6209, 262.8189) -> (-191.0513, 261.0508)
  line L426 (-191.0513, 261.0508) -> (-190.0684, 259.6997)
  line L427 (-190.0684, 259.6997) -> (-187.8018, 261.3485)
  line L428 (-187.8018, 261.3485) -> (-187.3773, 260.7649)
  line L429 (-187.3773, 260.7649) -> (-189.6438, 259.1161)
  line L430 (-189.6438, 259.1161) -> (-188.3119, 257.2852)
  line L431 (-188.3119, 257.2852) -> (-185.8815, 259.0533)
  line L432 (-185.8815, 259.0533) -> (-185.4569, 258.4697)
  line L433 (-185.4569, 258.4697) -> (-188.5429, 256.2247)
  line L434 (-184.8527, 265.4827) -> (-187.1708, 263.8464)
  line L435 (-187.1708, 263.8464) -> (-186.1788, 262.441)
  line L436 (-186.1788, 262.441) -> (-183.9576, 264.0089)
  line L437 (-183.9576, 264.0089) -> (-183.5414, 263.4193)
  line L438 (-183.5414, 263.4193) -> (-185.7626, 261.8514)
  line L439 (-185.7626, 261.8514) -> (-184.0693, 259.4525)
  line L440 (-184.0693, 259.4525) -> (-184.7316, 258.985)
  line L441 (-184.7316, 258.985) -> (-188.2493, 263.9685)
  line L442 (-188.2493, 263.9685) -> (-185.2689, 266.0723)
  line L443 (-185.2689, 266.0723) -> (-184.8527, 265.4827)
  line L444 (-181.6965, 261.1315) -> (-183.442, 267.3276)
  line L445 (-183.442, 267.3276) -> (-182.6178, 267.8912)
  line L446 (-182.6178, 267.8912) -> (-177.4772, 264.0165)
  line L447 (-177.4772, 264.0165) -> (-178.1831, 263.5338)
  line L448 (-178.1831, 263.5338) -> (-179.6028, 264.6291)
  line L449 (-179.6028, 264.6291) -> (-181.5247, 263.3149)
  line L450 (-181.5247, 263.3149) -> (-181.0191, 261.5946)
  line L451 (-181.0191, 261.5946) -> (-181.6965, 261.1315)
  line L452 (-180.177, 265.0748) -> (-182.5775, 266.9127)
  line L453 (-182.5775, 266.9127) -> (-181.7317, 264.0117)
  line L454 (-181.7317, 264.0117) -> (-180.177, 265.0748)
  line L455 (-173.2857, 266.7833) -> (-174.0451, 266.2827)
  line L456 (-174.0451, 266.2827) -> (-179.1936, 269.188)
  line L457 (-179.1936, 269.188) -> (-176.2984, 264.797)
  line L458 (-176.2984, 264.797) -> (-176.9298, 264.3806)
  line L459 (-176.9298, 264.3806) -> (-180.2876, 269.4733)
  line L460 (-180.2876, 269.4733) -> (-179.326, 270.1073)
  line L461 (-179.326, 270.1073) -> (-174.6165, 267.4276)
  line L462 (-174.6165, 267.4276) -> (-177.2749, 271.4597)
  line L463 (-177.2749, 271.4597) -> (-176.6435, 271.876)
  line L464 (-176.6435, 271.876) -> (-173.2857, 266.7833)
  line L465 (-170.4543, 268.595) -> (-172.4446, 267.3215)
  line L466 (-172.4446, 267.3215) -> (-172.7803, 267.8461)
  line L467 (-172.7803, 267.8461) -> (-172.1266, 268.2644)
  line L468 (-172.1266, 268.2644) -> (-174.7428, 272.3534)
  line L469 (-174.7428, 272.3534) -> (-175.3965, 271.9351)
  line L470 (-175.3965, 271.9351) -> (-175.7322, 272.4597)
  line L471 (-175.7322, 272.4597) -> (-173.7419, 273.7332)
  line L472 (-173.7419, 273.7332) -> (-173.4062, 273.2086)
  line L473 (-173.4062, 273.2086) -> (-174.0599, 272.7903)
  line L474 (-174.0599, 272.7903) -> (-171.4437, 268.7013)
  line L475 (-171.4437, 268.7013) -> (-170.79, 269.1196)
  line L476 (-170.79, 269.1196) -> (-170.4543, 268.595)
  spline S371 degree 2 poles (-167.1276, 274.2593) (-166.6871, 273.5495) (-166.5537, 272.0499) (-166.8387, 271.431) knots 0 0 0 1 2 2 2
  spline S372 degree 2 poles (-166.8387, 271.431) (-167.0798, 270.9381) (-167.7862, 270.2671) (-168.4163, 269.8762) knots 0 0 0 1 2 2 2
  line L477 (-168.4163, 269.8762) -> (-169.6092, 269.136)
  line L478 (-169.6092, 269.136) -> (-172.8253, 274.3194)
  line L479 (-172.8253, 274.3194) -> (-171.6449, 275.0517)
  spline S373 degree 2 poles (-171.6449, 275.0517) (-170.9141, 275.5052) (-169.9468, 275.8028) (-169.5329, 275.792) knots 0 0 0 1 2 2 2
  spline S374 degree 2 poles (-169.5329, 275.792) (-168.8272, 275.7703) (-167.5967, 275.0154) (-167.1276, 274.2593) knots 0 0 0 1 2 2 2
  spline S375 degree 2 poles (-167.8511, 273.8221) (-168.2212, 274.4185) (-169.1398, 275.0178) (-169.679, 275.0149) knots 0 0 0 1 2 2 2
  spline S376 degree 2 poles (-169.679, 275.0149) (-170.0579, 275.0067) (-170.775, 274.7654) (-171.2412, 274.4761) knots 0 0 0 1 2 2 2
  line L480 (-171.2412, 274.4761) -> (-171.7663, 274.1503)
  line L481 (-171.7663, 274.1503) -> (-169.2904, 270.1599)
  line L482 (-169.2904, 270.1599) -> (-168.7653, 270.4857)
  spline S377 degree 2 poles (-168.7653, 270.4857) (-168.3075, 270.7698) (-167.7056, 271.3468) (-167.5467, 271.7188) knots 0 0 0 1 2 2 2
  spline S378 degree 2 poles (-167.5467, 271.7188) (-167.3366, 272.1866) (-167.4758, 273.2172) (-167.8511, 273.8221) knots 0 0 0 1 2 2 2
  line L483 (-162.9439, 273.2164) -> (-164.9688, 271.9986)
  line L484 (-164.9688, 271.9986) -> (-165.2898, 272.5324)
  line L485 (-165.2898, 272.5324) -> (-164.6247, 272.9323)
  line L486 (-164.6247, 272.9323) -> (-167.1266, 277.0922)
  line L487 (-167.1266, 277.0922) -> (-167.7916, 276.6923)
  line L488 (-167.7916, 276.6923) -> (-168.1127, 277.226)
  line L489 (-168.1127, 277.226) -> (-166.0878, 278.4438)
  line L490 (-166.0878, 278.4438) -> (-165.7668, 277.9101)
  line L491 (-165.7668, 277.9101) -> (-166.4318, 277.5101)
  line L492 (-166.4318, 277.5101) -> (-163.93, 273.3502)
  line L493 (-163.93, 273.3502) -> (-163.2649, 273.7502)
  line L494 (-163.2649, 273.7502) -> (-162.9439, 273.2164)
  spline S379 degree 2 poles (-160.5597, 274.4958) (-161.1315, 274.1614) (-162.0735, 273.9311) (-162.5274, 273.8947) knots 0 0 0 1 2 2 2
  line L495 (-162.5274, 273.8947) -> (-163.0415, 274.7737)
  line L496 (-163.0415, 274.7737) -> (-162.9903, 274.8036)
  spline S380 degree 2 poles (-162.9903, 274.8036) (-162.455, 274.6815) (-161.3707, 274.8347) (-160.9653, 275.0717) knots 0 0 0 1 2 2 2
  spline S381 degree 2 poles (-160.9653, 275.0717) (-160.385, 275.4111) (-160.0738, 276.2402) (-160.3059, 276.6371) knots 0 0 0 1 2 2 2
  spline S382 degree 2 poles (-160.3059, 276.6371) (-160.4906, 276.9528) (-161.0317, 277.1632) (-161.4262, 277.0642) knots 0 0 0 1 2 2 2
  spline S383 degree 2 poles (-161.4262, 277.0642) (-161.7094, 276.9902) (-162.1696, 276.847) (-162.5175, 276.7466) knots 0 0 0 1 2 2 2
  spline S384 degree 2 poles (-162.5175, 276.7466) (-162.833, 276.6595) (-163.3913, 276.625) (-163.66, 276.7026) knots 0 0 0 1 2 2 2
  spline S385 degree 2 poles (-163.66, 276.7026) (-163.9245, 276.7828) (-164.3782, 277.1473) (-164.5579, 277.4545) knots 0 0 0 1 2 2 2
  spline S386 degree 2 poles (-164.5579, 277.4545) (-164.9322, 278.0946) (-164.4404, 279.5448) (-163.668, 279.9965) knots 0 0 0 1 2 2 2
  spline S387 degree 2 poles (-163.668, 279.9965) (-163.2242, 280.256) (-162.3368, 280.5403) (-161.9024, 280.571) knots 0 0 0 1 2 2 2
  line L497 (-161.9024, 280.571) -> (-161.4132, 279.7347)
  line L498 (-161.4132, 279.7347) -> (-161.4644, 279.7047)
  spline S388 degree 2 poles (-161.4644, 279.7047) (-161.8509, 279.7879) (-162.8357, 279.6701) (-163.2667, 279.418) knots 0 0 0 1 2 2 2
  spline S389 degree 2 poles (-163.2667, 279.418) (-163.7532, 279.1335) (-164.0878, 278.3251) (-163.8707, 277.9538) knots 0 0 0 1 2 2 2
  spline S390 degree 2 poles (-163.8707, 277.9538) (-163.676, 277.621) (-163.0897, 277.4313) (-162.7045, 277.5363) knots 0 0 0 1 2 2 2
  spline S391 degree 2 poles (-162.7045, 277.5363) (-162.4477, 277.6064) (-161.7135, 277.8296) (-161.4627, 277.8904) knots 0 0 0 1 2 2 2
  spline S392 degree 2 poles (-161.4627, 277.8904) (-160.8235, 278.0409) (-159.9282, 277.6655) (-159.6412, 277.1747) knots 0 0 0 1 2 2 2
  spline S393 degree 2 poles (-159.6412, 277.1747) (-159.459, 276.8632) (-159.3613, 276.1186) (-159.4652, 275.7773) knots 0 0 0 1 2 2 2
  spline S394 degree 2 poles (-159.4652, 275.7773) (-159.5822, 275.3996) (-160.0775, 274.7778) (-160.5597, 274.4958) knots 0 0 0 1 2 2 2
  spline S395 degree 2 poles (-153.505, 280.8891) (-153.2772, 280.4785) (-153.1635, 279.6315) (-153.2631, 279.2709) knots 0 0 0 1 2 2 2
  spline S396 degree 2 poles (-153.2631, 279.2709) (-153.3642, 278.8927) (-153.8193, 278.3067) (-154.1781, 278.1077) knots 0 0 0 1 2 2 2
  spline S397 degree 2 poles (-154.1781, 278.1077) (-154.5369, 277.9087) (-155.2634, 277.8223) (-155.6224, 277.9397) knots 0 0 0 1 2 2 2
  spline S398 degree 2 poles (-155.6224, 277.9397) (-156.0597, 278.0758) (-156.9105, 278.8758) (-157.3037, 279.5847) knots 0 0 0 1 2 2 2
  spline S399 degree 2 poles (-157.3037, 279.5847) (-157.6898, 280.2807) (-158.0255, 281.5586) (-157.9574, 282.139) knots 0 0 0 1 2 2 2
  spline S400 degree 2 poles (-157.9574, 282.139) (-157.8932, 282.706) (-157.2285, 283.6682) (-156.6277, 284.0015) knots 0 0 0 1 2 2 2
  spline S401 degree 2 poles (-156.6277, 284.0015) (-156.4504, 284.0998) (-156.12, 284.2379) (-155.9817, 284.2637) knots 0 0 0 1 2 2 2
  line L499 (-155.9817, 284.2637) -> (-155.6004, 283.5764)
  line L500 (-155.6004, 283.5764) -> (-155.6307, 283.5596)
  spline S402 degree 2 poles (-155.6307, 283.5596) (-155.7589, 283.5563) (-156.1724, 283.4457) (-156.3799, 283.3306) knots 0 0 0 1 2 2 2
  spline S403 degree 2 poles (-156.3799, 283.3306) (-157.0456, 282.9614) (-157.3638, 281.609) (-156.9525, 280.684) knots 0 0 0 1 2 2 2
  spline S404 degree 2 poles (-156.9525, 280.684) (-156.7958, 281.0027) (-156.3676, 281.4946) (-156.0478, 281.672) knots 0 0 0 1 2 2 2
  spline S405 degree 2 poles (-156.0478, 281.672) (-155.7365, 281.8447) (-155.2001, 281.9783) (-154.8396, 281.9295) knots 0 0 0 1 2 2 2
  spline S406 degree 2 poles (-154.8396, 281.9295) (-154.4233, 281.8721) (-153.7592, 281.3474) (-153.505, 280.8891) knots 0 0 0 1 2 2 2
  spline S407 degree 2 poles (-154.2145, 280.4561) (-154.3967, 280.7846) (-154.8166, 281.1339) (-155.0931, 281.184) knots 0 0 0 1 2 2 2
  spline S408 degree 2 poles (-155.0931, 281.184) (-155.2981, 281.2173) (-155.6933, 281.0942) (-155.8792, 280.9911) knots 0 0 0 1 2 2 2
  spline S409 degree 2 poles (-155.8792, 280.9911) (-156.1299, 280.852) (-156.5172, 280.4393) (-156.6672, 280.1696) knots 0 0 0 1 2 2 2
  spline S410 degree 2 poles (-156.6672, 280.1696) (-156.6283, 280.0894) (-156.5554, 279.9376) (-156.4931, 279.8252) knots 0 0 0 1 2 2 2
  spline S411 degree 2 poles (-156.4931, 279.8252) (-156.1862, 279.2719) (-155.5936, 278.7131) (-155.331, 278.627) knots 0 0 0 1 2 2 2
  spline S412 degree 2 poles (-155.331, 278.627) (-155.0862, 278.5423) (-154.6833, 278.5906) (-154.4975, 278.6937) knots 0 0 0 1 2 2 2
  spline S413 degree 2 poles (-154.4975, 278.6937) (-154.0652, 278.9335) (-153.874, 279.8422) (-154.2145, 280.4561) knots 0 0 0 1 2 2 2
  spline S414 degree 2 poles (-153.0695, 285.1488) (-153.2655, 285.0437) (-153.6019, 284.74) (-153.7495, 284.5655) knots 0 0 0 1 2 2 2
  spline S415 degree 2 poles (-153.7495, 284.5655) (-153.8841, 284.398) (-154.0571, 284.1034) (-154.1199, 283.9799) knots 0 0 0 1 2 2 2
  line L501 (-154.1199, 283.9799) -> (-154.1635, 283.9566)
  line L502 (-154.1635, 283.9566) -> (-154.5722, 284.719)
  spline S416 degree 2 poles (-154.5722, 284.719) (-154.4046, 284.9715) (-153.7084, 285.6083) (-153.3468, 285.8021) knots 0 0 0 1 2 2 2
  spline S417 degree 2 poles (-153.3468, 285.8021) (-152.9808, 285.9983) (-152.3568, 286.1421) (-152.0505, 286.1044) knots 0 0 0 1 2 2 2
  spline S418 degree 2 poles (-152.0505, 286.1044) (-151.7242, 286.0605) (-151.2163, 285.699) (-151.0388, 285.3679) knots 0 0 0 1 2 2 2
  spline S419 degree 2 poles (-151.0388, 285.3679) (-150.8006, 284.9235) (-151.0248, 283.9396) (-151.3876, 283.6329) knots 0 0 0 1 2 2 2
  line L503 (-151.3876, 283.6329) -> (-151.3596, 283.5807)
  spline S420 degree 2 poles (-151.3596, 283.5807) (-151.171, 283.6369) (-150.6992, 283.6879) (-150.4495, 283.6198) knots 0 0 0 1 2 2 2
  spline S421 degree 2 poles (-150.4495, 283.6198) (-150.2022, 283.556) (-149.7315, 283.1802) (-149.5424, 282.8273) knots 0 0 0 1 2 2 2
  spline S422 degree 2 poles (-149.5424, 282.8273) (-149.3485, 282.4656) (-149.2676, 281.7182) (-149.368, 281.3615) knots 0 0 0 1 2 2 2
  spline S423 degree 2 poles (-149.368, 281.3615) (-149.4725, 280.9914) (-150.0037, 280.3814) (-150.4263, 280.1549) knots 0 0 0 1 2 2 2
  spline S424 degree 2 poles (-150.4263, 280.1549) (-150.8315, 279.9377) (-151.7295, 279.7087) (-152.072, 279.699) knots 0 0 0 1 2 2 2
  line L504 (-152.072, 279.699) -> (-152.4807, 280.4614)
  line L505 (-152.4807, 280.4614) -> (-152.4284, 280.4894)
  spline S425 degree 2 poles (-152.4284, 280.4894) (-152.1131, 280.4453) (-151.1829, 280.5514) (-150.8038, 280.7545) knots 0 0 0 1 2 2 2
  spline S426 degree 2 poles (-150.8038, 280.7545) (-150.5816, 280.8736) (-150.2119, 281.2513) (-150.1502, 281.4919) knots 0 0 0 1 2 2 2
  spline S427 degree 2 poles (-150.1502, 281.4919) (-150.0929, 281.7301) (-150.1459, 282.1953) (-150.3023, 282.4872) knots 0 0 0 1 2 2 2
  spline S428 degree 2 poles (-150.3023, 282.4872) (-150.4588, 282.7791) (-150.8319, 283.0671) (-151.0428, 283.0943) knots 0 0 0 1 2 2 2
  spline S429 degree 2 poles (-151.0428, 283.0943) (-151.2537, 283.1214) (-151.7119, 282.9824) (-151.9559, 282.8516) knots 0 0 0 1 2 2 2
  line L506 (-151.9559, 282.8516) -> (-152.2609, 282.6881)
  line L507 (-152.2609, 282.6881) -> (-152.5808, 283.285)
  line L508 (-152.5808, 283.285) -> (-152.3412, 283.4134)
  spline S430 degree 2 poles (-152.3412, 283.4134) (-151.8576, 283.6727) (-151.4952, 284.4614) (-151.7311, 284.9015) knots 0 0 0 1 2 2 2
  spline S431 degree 2 poles (-151.7311, 284.9015) (-151.8408, 285.1063) (-152.1541, 285.3141) (-152.3272, 285.3335) knots 0 0 0 1 2 2 2
  spline S432 degree 2 poles (-152.3272, 285.3335) (-152.5113, 285.3526) (-152.8821, 285.2492) (-153.0695, 285.1488) knots 0 0 0 1 2 2 2
  line L509 (-146.8558, 288.0276) -> (-146.8163, 282.209)
  line L510 (-146.8163, 282.209) -> (-147.5889, 281.8091)
  line L511 (-147.5889, 281.8091) -> (-147.5876, 287.8714)
  line L512 (-147.5876, 287.8714) -> (-150.3841, 286.4239)
  line L513 (-150.3841, 286.4239) -> (-150.7136, 287.0604)
  line L514 (-150.7136, 287.0604) -> (-147.2762, 288.8397)
  line L515 (-147.2762, 288.8397) -> (-146.8558, 288.0276)
  spline S433 degree 2 poles (-145.7967, 287.3685) (-146.0066, 287.7886) (-146.0814, 288.6243) (-145.9685, 288.9957) knots 0 0 0 1 2 2 2
  spline S434 degree 2 poles (-145.9685, 288.9957) (-145.8645, 289.3516) (-145.3403, 289.9505) (-145.0042, 290.1183) knots 0 0 0 1 2 2 2
  spline S435 degree 2 poles (-145.0042, 290.1183) (-144.6283, 290.3061) (-143.8922, 290.3589) (-143.5473, 290.2327) knots 0 0 0 1 2 2 2
  spline S436 degree 2 poles (-143.5473, 290.2327) (-143.1141, 290.0734) (-142.3186, 289.2551) (-141.9452, 288.5078) knots 0 0 0 1 2 2 2
  spline S437 degree 2 poles (-141.9452, 288.5078) (-141.6073, 287.8312) (-141.3071, 286.4671) (-141.4024, 285.9166) knots 0 0 0 1 2 2 2